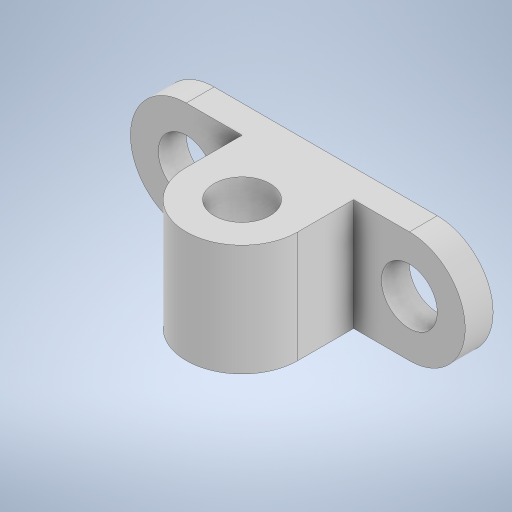
# Autodesk Inventor part: tarea 1
Saved by Autodesk Inventor 2024 (Build 280153000, 153)
## iProperties
Created: 2024-01-23
Part Number: tarea 1
Material: Genérico
Document SubType Name: Modeling
Designer: joseo
Density: 1 g/cm^3
Appearance: Valor por defecto
Author: joseo
Autodesk Inventor part; units mm, degrees
ref_plane "YZ Plane" through (0, 0, 0) normal (1, 0, 0) x (0, 1, 0)
ref_plane "XZ Plane" through (0, 0, 0) normal (0, 1, 0) x (-1, 0, 0)
ref_plane "XY Plane" through (0, 0, 0) normal (0, 0, 1) x (1, 0, 0)
sketch "Boceto1" plane through (0, 0, 0) normal (0, 0, 1) x (1, 0, 0)
  line L0 (40, -20) -> (-40, -20)
  line L1 (-40, -20) -> (-40, 20)
  line L2 (-40, 20) -> (40, 20)
  line L3 (40, 20) -> (40, -20)
  line L4 (40, -20) -> (-40, 20) construction
  line L5 (-40, -20) -> (40, 20) construction
  circle A0 centre (-40, 0) radius 10
  circle A1 centre (40, 0) radius 10
  arc A2 (-40, 20) -> (-40, -20) centre (-40, 0) ccw
  arc A3 (40, -20) -> (40, 20) centre (40, 0) ccw
  point P0 (0, 0)
  dimension "d0" = 80
  dimension "d1" = 40
  dimension "d2" = 20
  dimension "d3" = 20
  constraints: 12 end point, 4 centre point, 4 midpoint, 4 point on circle, 2 coincident, 2 parallel, 1 horizontal, 1 perpendicular
  measures "d0" distance of L1.end L2.end
  measures "d1" distance of L0.end L1.end
  measures "d2" diameter of A0
  measures "d3" diameter of A1
extrude "Extrusión1" add sketch "Boceto1" along normal blind 10 contours L0 L1 A0 L2 L3 A1 | L3 A1 A3 | A2 L1 A0
sketch "Boceto2" plane through (0, 0, 10) normal (0, 0, 1) x (1, 0, 0)
  line L0 (20, -20) -> (-20, -20)
  line L1 (-20, -20) -> (-20, 20)
  line L2 (-20, 20) -> (20, 20)
  line L3 (20, 20) -> (20, -20)
  line L4 (20, -20) -> (-20, 20) construction
  line L5 (-20, -20) -> (20, 20) construction
  point P0 (0, 0)
  dimension "d6" = 40
  dimension "d7" = 40
  constraints: 12 end point, 2 midpoint, 2 parallel, 1 horizontal, 1 perpendicular
  measures "d6" distance of L1.end L2.end
  measures "d7" distance of L0.end L1.end
extrude "Extrusión2" add sketch "Boceto2" along normal blind 20
sketch "Boceto4" plane through (-40, -20, 0) normal (0, -1, 0) x (1, 0, 0)
  line L0 (60, 30) -> (20, 30) projected
  arc A0 (60, 30) -> (20, 30) centre (40, 30) ccw
  point P0 (40, 0)
  point P1 (20, 70)
  constraints: 2 point on circle, 1 centre point, 1 midpoint
extrude "Extrusión4" add sketch "Boceto4" against normal blind 40
sketch "Boceto5" plane through (-40, -20, 0) normal (0, -1, 0) x (1, 0, 0)
  arc A0 (60, 30) -> (20, 30) centre (40, 30) ccw projected
  circle A1 centre (40, 30) radius 10
  point P0 (40, 0)
  dimension "d15" = 20
  constraints: 1 centre point, 1 coincident
  measures "d15" diameter of A1
extrude "Extrusión5" cut sketch "Boceto5" against normal blind 40
